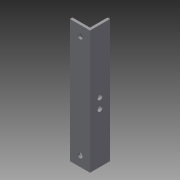
# Autodesk Inventor part: 1x1 angle support lengthwise
Saved by Autodesk Inventor 2015 (Build 190159000, 159)
## iProperties
Created: 2015-01-22
Part Number: 1x1 angle support lengthwise
Material: Generic
Document SubType Name: Modeling
Designer: 215152
Density: 1 g/cm^3
Appearance: Default
Author: 215152
Autodesk Inventor part; units mm, degrees
ref_plane "YZ Plane" through (0, 0, 0) normal (1, 0, 0) x (0, 1, 0)
ref_plane "XZ Plane" through (0, 0, 0) normal (0, 1, 0) x (-1, 0, 0)
ref_plane "XY Plane" through (0, 0, 0) normal (0, 0, 1) x (1, 0, 0)
sketch "Sketch1" plane through (0, 0, 0) normal (0, 1, 0) x (-1, 0, 0)
  line L0 (0, 0) -> (25.4, 0)
  line L1 (25.4, 0) -> (25.4, -3.175)
  line L2 (25.4, -3.175) -> (0, -3.175)
  line L3 (0, -3.175) -> (0, 0)
  line L4 (0, 0) -> (3.175, 0)
  line L5 (3.175, 0) -> (3.175, -25.4)
  line L6 (3.175, -25.4) -> (0, -25.4)
  line L7 (0, -25.4) -> (0, 0)
  dimension "d0" = 25.4
  dimension "d1" = 3.175
  dimension "d2" = 3.175
  dimension "d3" = 25.4
  constraints: 16 end point, 4 parallel, 2 horizontal, 2 perpendicular
  measures "d0" distance of L1.end L2.end
  measures "d1" distance of L0.end L1.end
  measures "d2" distance of L5.end L6.end
  measures "d3" distance of L4.end L5.end
extrude "Extrusion1" add sketch "Sketch1" along normal blind 155.575
sketch "Sketch2" plane through (0, 0, 0) normal (1, 0, 0) x (0, 0, -1)
  line L0 (0, 155.575) -> (25.4, 155.575) projected
  line L1 (0, 0) -> (0, 155.575) projected
  line L2 (0, 0) -> (25.4, 0) projected
  line L3 (25.4, 0) -> (25.4, 155.575) projected
  point P0 (12.7, 63.5)
  point P1 (12.7, 76.2)
  dimension "d6" = 12.7
  dimension "d7" = 12.7
  dimension "d8" = 63.5
  dimension "d9" = 79.375
  measures "d6" distance from line of L1 point (12.7, 63.5)
  measures "d7" distance from line of L1 point (12.7, 76.2)
  measures "d8" distance from line of L2 point (12.7, 63.5)
  measures "d9" distance from line of L0 point (12.7, 76.2)
hole "Hole1" at (0, 63.5, -12.7) at (0, 76.2, -12.7) direction (-1, 0, 0) diameter 6.35 end through all
sketch "Sketch3" plane through (-25.4, 0, 0) normal (0, 0, 1) x (1, 0, 0)
  line L0 (0, 0) -> (25.4, 0) projected
  line L1 (25.4, 0) -> (25.4, 155.575) projected
  line L2 (0, 155.575) -> (25.4, 155.575) projected
  line L3 (0, 0) -> (0, 155.575) projected
  point P0 (12.7, 12.7)
  point P1 (12.7, 142.875)
  dimension "d17" = 12.7
  dimension "d18" = 12.7
  dimension "d19" = 12.7
  dimension "d20" = 12.7
  measures "d17" distance from line of L3 point (12.7, 12.7)
  measures "d18" distance from line of L0 point (12.7, 12.7)
  measures "d19" distance from line of L2 point (12.7, 142.875)
  measures "d20" distance from line of L3 point (12.7, 142.875)
hole "Hole2" at (-12.7, 12.7, 0) at (-12.7, 142.875, 0) direction (0, 0, -1) diameter 6.35 end through all
body "Solid1"
